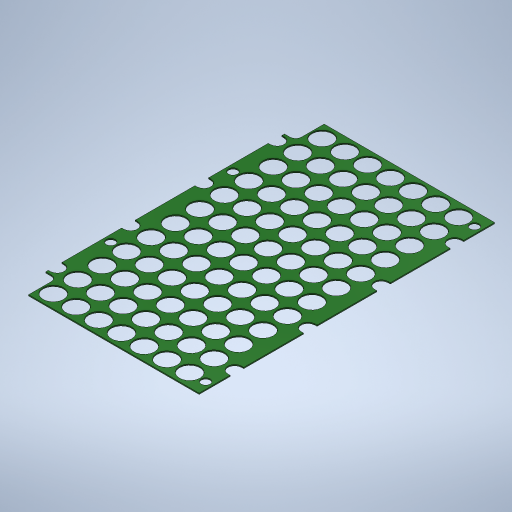
# Autodesk Inventor part: PCB
Saved by Autodesk Inventor 2024 (Build 280153000, 153)
## iProperties
Created: 2025-03-26
Part Number: PCB
Material: PC/ABS-Kunststoff
Document SubType Name: Modeling
Designer: David Lill
Density: 0.357273 g/cm^3
Appearance: Glatt - Waldgrün
Author: David Lill
Autodesk Inventor part; units mm, degrees
ref_plane "YZ Plane" through (0, 0, 0) normal (1, 0, 0) x (0, 1, 0)
ref_plane "XZ Plane" through (0, 0, 0) normal (0, 1, 0) x (-1, 0, 0)
ref_plane "XY Plane" through (0, 0, 0) normal (0, 0, 1) x (1, 0, 0)
sketch "Skizze3" plane through (0, 0, 0) normal (0, 0, 1) x (1, 0, 0)
  line L0 (0, 0) -> (0, 260)
  arc A0 (-2, 168.25) -> (-2, 156.25) centre (-2, 162.25) ccw
  line L1 (-2, 156.25) -> (0, 156.25)
  line L2 (0, 0) -> (0, 260)
  arc A1 (-2, 232.75) -> (-2, 220.75) centre (-2, 226.75) ccw
  line L3 (-2, 220.75) -> (0, 220.75)
  line L4 (0, 130) -> (-160, 130)
  line L5 (0, 260) -> (-160, 260)
  line L6 (-80, 260) -> (-80, 0)
  line L7 (-159.8953, 260) -> (-159.8953, 0)
  line L8 (-160, 0) -> (0, 0)
  line L9 (0, 0) -> (-160, 0)
  line L10 (-16.9586, 239.25) -> (-9, 239.25)
  arc A2 (-9, 239.25) -> (-9, 257.25) centre (-9, 248.25) ccw
  line L11 (-9, 257.25) -> (-16.9586, 257.25)
  arc A3 (-16.9586, 239.25) -> (-16.9586, 257.25) centre (-20, 248.25) ccw
  line L12 (-143.0414, 85.25) -> (-151, 85.25)
  arc A4 (-151, 85.25) -> (-151, 67.25) centre (-151, 76.25) ccw
  line L13 (-151, 67.25) -> (-143.0414, 67.25)
  arc A5 (-143.0414, 85.25) -> (-143.0414, 67.25) centre (-140, 76.25) ccw
  line L14 (-151, 174.75) -> (-143.0414, 174.75)
  arc A6 (-143.0414, 192.75) -> (-143.0414, 174.75) centre (-140, 183.75) ccw
  line L15 (-143.0414, 192.75) -> (-151, 192.75)
  arc A7 (-151, 192.75) -> (-151, 174.75) centre (-151, 183.75) ccw
  line L16 (-9, 20.75) -> (-16.9586, 20.75)
  arc A8 (-16.9586, 2.75) -> (-16.9586, 20.75) centre (-20, 11.75) ccw
  line L17 (-16.9586, 2.75) -> (-9, 2.75)
  arc A9 (-9, 2.75) -> (-9, 20.75) centre (-9, 11.75) ccw
  line L18 (-150, 0) -> (-150, 20)
  line L19 (-160, 25) -> (-155, 25)
  arc A10 (-150, 20) -> (-155, 25) centre (-155, 20) ccw
  line L20 (-150, 260) -> (-150, 240)
  line L21 (-160, 235) -> (-155, 235)
  arc A11 (-155, 235) -> (-150, 240) centre (-155, 240) ccw
  line L22 (0, 232.75) -> (-2, 232.75)
  arc A12 (-2, 232.75) -> (-2, 220.75) centre (-2, 226.75) ccw
  line L23 (-2, 220.75) -> (0, 220.75)
  line L24 (0, 168.25) -> (-2, 168.25)
  arc A13 (-2, 168.25) -> (-2, 156.25) centre (-2, 162.25) ccw
  line L25 (-2, 156.25) -> (0, 156.25)
  line L26 (-160, 156.25) -> (-158, 156.25)
  arc A14 (-158, 156.25) -> (-158, 168.25) centre (-158, 162.25) ccw
  line L27 (-158, 168.25) -> (-160, 168.25)
  line L28 (0, 39.25) -> (-2, 39.25)
  arc A15 (-2, 39.25) -> (-2, 27.25) centre (-2, 33.25) ccw
  line L29 (-2, 27.25) -> (0, 27.25)
  line L30 (0, 91.75) -> (-2, 91.75)
  arc A16 (-2, 103.75) -> (-2, 91.75) centre (-2, 97.75) ccw
  line L31 (-2, 103.75) -> (0, 103.75)
  line L32 (-160, 91.75) -> (-158, 91.75)
  arc A17 (-158, 91.75) -> (-158, 103.75) centre (-158, 97.75) ccw
  line L33 (-158, 103.75) -> (-160, 103.75)
  line L34 (-160, 27.25) -> (-158, 27.25)
  arc A18 (-158, 27.25) -> (-158, 39.25) centre (-158, 33.25) ccw
  line L35 (-158, 39.25) -> (-160, 39.25)
  line L36 (-160, 232.75) -> (-158, 232.75)
  arc A19 (-158, 220.75) -> (-158, 232.75) centre (-158, 226.75) ccw
  line L37 (-158, 220.75) -> (-160, 220.75)
  circle A20 centre (-20, 226.75) radius 9
  circle A21 centre (-20, 248.25) radius 9
  circle A22 centre (-20, 205.25) radius 9
  circle A23 centre (-20, 162.25) radius 9
  circle A24 centre (-20, 119.25) radius 9
  circle A25 centre (-20, 76.25) radius 9
  circle A26 centre (-20, 33.25) radius 9
  circle A27 centre (-20, 11.75) radius 9
  circle A28 centre (-20, 54.75) radius 9
  circle A29 centre (-20, 97.75) radius 9
  circle A30 centre (-20, 140.75) radius 9
  circle A31 centre (-20, 183.75) radius 9
  circle A32 centre (-40, 226.75) radius 9
  circle A33 centre (-40, 248.25) radius 9
  circle A34 centre (-40, 205.25) radius 9
  circle A35 centre (-40, 162.25) radius 9
  circle A36 centre (-40, 119.25) radius 9
  circle A37 centre (-40, 76.25) radius 9
  circle A38 centre (-40, 33.25) radius 9
  circle A39 centre (-40, 11.75) radius 9
  circle A40 centre (-40, 54.75) radius 9
  circle A41 centre (-40, 97.75) radius 9
  circle A42 centre (-40, 140.75) radius 9
  circle A43 centre (-40, 183.75) radius 9
  circle A44 centre (-60, 226.75) radius 9
  circle A45 centre (-60, 248.25) radius 9
  circle A46 centre (-60, 205.25) radius 9
  circle A47 centre (-60, 162.25) radius 9
  circle A48 centre (-60, 119.25) radius 9
  circle A49 centre (-60, 76.25) radius 9
  circle A50 centre (-60, 33.25) radius 9
  circle A51 centre (-60, 11.75) radius 9
  circle A52 centre (-60, 54.75) radius 9
  circle A53 centre (-60, 97.75) radius 9
  circle A54 centre (-60, 140.75) radius 9
  circle A55 centre (-60, 183.75) radius 9
  circle A56 centre (-80, 226.75) radius 9
  circle A57 centre (-80, 248.25) radius 9
  circle A58 centre (-80, 205.25) radius 9
  circle A59 centre (-80, 162.25) radius 9
  circle A60 centre (-80, 119.25) radius 9
  circle A61 centre (-80, 76.25) radius 9
  circle A62 centre (-80, 33.25) radius 9
  circle A63 centre (-80, 11.75) radius 9
  circle A64 centre (-80, 54.75) radius 9
  circle A65 centre (-80, 97.75) radius 9
  circle A66 centre (-80, 140.75) radius 9
  circle A67 centre (-80, 183.75) radius 9
  circle A68 centre (-100, 226.75) radius 9
  circle A69 centre (-100, 248.25) radius 9
  circle A70 centre (-100, 205.25) radius 9
  circle A71 centre (-100, 162.25) radius 9
  circle A72 centre (-100, 119.25) radius 9
  circle A73 centre (-100, 76.25) radius 9
  circle A74 centre (-100, 33.25) radius 9
  circle A75 centre (-100, 11.75) radius 9
  circle A76 centre (-100, 54.75) radius 9
  circle A77 centre (-100, 97.75) radius 9
  circle A78 centre (-100, 140.75) radius 9
  circle A79 centre (-100, 183.75) radius 9
  circle A80 centre (-120, 226.75) radius 9
  circle A81 centre (-120, 248.25) radius 9
  circle A82 centre (-120, 205.25) radius 9
  circle A83 centre (-120, 162.25) radius 9
  circle A84 centre (-120, 119.25) radius 9
  circle A85 centre (-120, 76.25) radius 9
  circle A86 centre (-120, 33.25) radius 9
  circle A87 centre (-120, 11.75) radius 9
  circle A88 centre (-120, 54.75) radius 9
  circle A89 centre (-120, 97.75) radius 9
  circle A90 centre (-120, 140.75) radius 9
  circle A91 centre (-120, 183.75) radius 9
  circle A92 centre (-140, 226.75) radius 9
  circle A93 centre (-140, 183.75) radius 9
  circle A94 centre (-140, 140.75) radius 9
  circle A95 centre (-140, 97.75) radius 9
  circle A96 centre (-140, 54.75) radius 9
  circle A97 centre (-140, 11.75) radius 9
  circle A98 centre (-140, 33.25) radius 9
  circle A99 centre (-140, 76.25) radius 9
  circle A100 centre (-140, 119.25) radius 9
  circle A101 centre (-140, 162.25) radius 9
  circle A102 centre (-140, 205.25) radius 9
  circle A103 centre (-140, 248.25) radius 9
  line L38 (0, 0) -> (0, 260)
  line L39 (-160, 0) -> (0, 0)
  line L40 (-159.8953, 260) -> (-159.8953, 0)
  line L41 (-160, 0) -> (0, 0)
  line L42 (0, 260) -> (-160, 260)
  line L43 (0, 130) -> (-160, 130)
  circle A104 centre (-20, 11.75) radius 9
  circle A105 centre (-154, 76.25) radius 4
  circle A106 centre (-154, 183.75) radius 4
  line L44 (-80, 260) -> (-80, 0)
  circle A107 centre (-6, 11.75) radius 4
  circle A108 centre (-6, 248.25) radius 4
  circle A109 centre (-20, 76.25) radius 9
  circle A110 centre (-20, 76.25) radius 9
  line L45 (-156.8953, 69) -> (-149.8953, 69)
  line L46 (-149.8953, 69) -> (-149.8953, 62)
  line L47 (-149.8953, 62) -> (-156.8953, 62)
  line L48 (-156.8953, 62) -> (-156.8953, 69)
  point P0 (-155, 235)
  point P1 (-158, 220.75)
  point P2 (-158, 168.25)
  point P3 (-158, 156.25)
  point P4 (-158, 103.75)
  point P5 (-158, 91.75)
  point P6 (-158, 39.25)
  point P7 (-158, 27.25)
  point P8 (-150, 0)
  point P9 (0, 27.25)
  point P10 (-2, 27.25)
  point P11 (-2, 39.25)
  point P12 (0, 39.25)
  point P13 (-2, 91.75)
  point P14 (-2, 103.75)
  point P15 (0, 103.75)
  point P16 (-2, 156.25)
  point P17 (-2, 168.25)
  point P18 (-2, 220.75)
  point P19 (-2, 232.75)
  point P20 (-159.8953, 235)
  point P21 (-159.8953, 232.75)
  point P22 (-159.8953, 220.75)
  point P23 (-159.8953, 168.25)
  point P24 (-159.8953, 156.25)
  point P25 (-159.8953, 103.75)
  point P26 (-159.8953, 91.75)
  point P27 (-159.8953, 39.25)
  point P28 (-159.8953, 27.25)
  point P29 (-159.8953, 25)
  point P30 (-149.8953, 65.5)
  dimension "d49" = 7
  dimension "d50" = 3
  dimension "d51" = 10.75
  constraints: 111 centre point, 98 end point, 41 point on circle, 37 horizontal, 11 vertical, 2 parallel, 2 perpendicular, 1 midpoint, 352 other
  measures "d49" distance of L46.end L47.end
  measures "d50" distance between parallel lines of L7 L48
  measures "d51" vertical distance of A5.centre point (-149.895, 65.5)
extrude "Extrusion3" add sketch "Skizze3" along normal blind 1 contours A9 L17 A8 L16 | L0 L8 L6 A63 A62 A64 A61 A65 A60 L4 L31 A16 L30 L28 A15 L29 | L8 L18 A10 L19 L7 L34 A18 L35 A4 L45 L48 L47 L46 L13 A5 L12 L32 A17 L33 L4 L6 A60 A65 A61 A64 A62 A63 | A2 L10 A3 L11 | L4 L6 A66 A59 A67 A58 A56 A57 L5 L0 L22 A1 L3 L24 A0 L1 | L4 L7 L26 A14 L27 A7 L14 A6 L15 L37 A19 L36 L21 A11 L20 L5 L6 A57 A56 A58 A67 A59 A66 | L7 A7 L15 A6 L14 | A4 L12 A5 L13 L46 L45 L7 | L45 L46 L13 A4 | A4 L13 L46 L47 L48 L45
